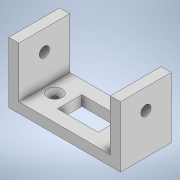
# Autodesk Inventor part: 2nd to 3rd arm linking clamp
Saved by Autodesk Inventor 2022 (Build 260153000, 153)
## iProperties
Created: 2021-06-29
Part Number: 2nd to 3rd arm linking clamp
Material: Generic
Document SubType Name: Modeling
Designer: USER
Density: 1 g/cm^3
Appearance: Default
Author: USER
Autodesk Inventor part; units mm, degrees
ref_plane "YZ Plane" through (0, 0, 0) normal (1, 0, 0) x (0, 1, 0)
ref_plane "XZ Plane" through (0, 0, 0) normal (0, 1, 0) x (-1, 0, 0)
ref_plane "XY Plane" through (0, 0, 0) normal (0, 0, 1) x (1, 0, 0)
sketch "Sketch1" plane through (0, 0, 0) normal (0, 0, 1) x (1, 0, 0)
  line L0 (0, 0) -> (55, 0)
  line L1 (55, 0) -> (55, 30)
  line L2 (55, 30) -> (50, 30)
  line L3 (50, 30) -> (50, 5)
  line L4 (50, 5) -> (5, 5)
  line L5 (5, 5) -> (5, 30)
  line L6 (5, 30) -> (0, 30)
  line L7 (0, 30) -> (0, 0)
  dimension "d0" = 55
  dimension "d1" = 30
  dimension "d2" = 5
  dimension "d3" = 25
  dimension "d4" = 45
  dimension "d5" = 25
  dimension "d6" = 5
  constraints: 16 end point, 3 perpendicular, 2 point on line, 1 horizontal, 1 vertical
  measures "d0" distance of L0.start L0.end
  measures "d1" distance of L0.end L1.end
  measures "d2" distance of L1.end L2.end
  measures "d3" distance of L2.end L3.end
  measures "d4" distance of L3.end L4.end
  measures "d5" distance of L4.end L5.end
  measures "d6" distance of L5.end L6.end
extrude "Extrusion1" add sketch "Sketch1" along normal blind 25
sketch "Sketch2" plane through (55, 0, 0) normal (1, 0, 0) x (0, 0, -1)
  circle A0 centre (-12.5, 20) radius 2.5
  line L0 (0, 30) -> (-25, 30) projected
  line L1 (0, 0) -> (0, 30) projected
  dimension "d9" = 5
  dimension "d10" = 10
  dimension "d11" = 12.5
  constraints: 1 centre point
  measures "d9" diameter of A0
  measures "d10" distance from line of L0 A0.centre
  measures "d11" distance from line of L1 A0.centre
extrude "Extrusion2" cut sketch "Sketch2" against normal through all
sketch "Sketch3" plane through (5, 5, 0) normal (0, 1, 0) x (1, 0, 0)
  line L0 (12.5, -6.5) -> (32.5, -6.5)
  line L1 (32.5, -6.5) -> (32.5, -18.5)
  line L2 (32.5, -18.5) -> (12.5, -18.5)
  line L3 (12.5, -18.5) -> (12.5, -6.5)
  line L4 (12.5, -6.5) -> (32.5, -18.5) construction
  line L5 (32.5, -6.5) -> (12.5, -18.5) construction
  line L6 (45, 0) -> (0, 0) projected
  line L7 (0, 0) -> (0, -25) projected
  point P0 (-5, 0)
  point P1 (22.5, -12.5)
  dimension "d14" = 20
  dimension "d15" = 12
  dimension "d16" = 12.5
  dimension "d17" = 22.5
  constraints: 12 end point, 2 midpoint, 2 parallel, 1 horizontal, 1 perpendicular
  measures "d14" distance of L1.end L2.end
  measures "d15" distance of L0.end L1.end
  measures "d16" distance from line of L6 point (22.5, -12.5)
  measures "d17" distance from line of L7 point (22.5, -12.5)
extrude "Extrusion3" cut sketch "Sketch3" against normal through all
sketch "Sketch4" plane through (5, 5, 0) normal (0, 1, 0) x (1, 0, 0)
  circle A0 centre (5.25, -12.5) radius 3.625
  circle A1 centre (39.75, -12.5) radius 3.625
  line L0 (0, -10) -> (0, -15) projected
  line L1 (45, 0) -> (45, -25) projected
  line L2 (45, -25) -> (0, -25) projected
  point P0 (-5, 0)
  dimension "d20" = 7.25
  dimension "d21" = 7.25
  dimension "d22" = 5.25
  dimension "d23" = 5.25
  dimension "d24" = 12.5
  dimension "d25" = 12.5
  constraints: 2 centre point
  measures "d20" diameter of A0
  measures "d21" diameter of A1
  measures "d22" distance from line of L0 A0.centre
  measures "d23" distance from line of L1 A1.centre
  measures "d24" distance from line of L2 A0.centre
  measures "d25" distance from line of L2 A1.centre
extrude "Extrusion4" cut sketch "Sketch4" against normal blind 2.1735 draft -45
sketch "Sketch5" plane through (10.25, 2.8265, 12.5) normal (0, 1, 0) x (1, 0, 0)
  circle A0 centre (0, 0) radius 1.4515
  circle A1 centre (34.5, 0) radius 1.4515
  line L0 (39.75, 12.5) -> (39.75, -12.5) projected
  point P0 (-10.25, 12.5)
  dimension "d28" = 2.903
  dimension "d29" = 2.903
  dimension "d30" = 5.25
  constraints: 2 centre point
  measures "d28" diameter of A0
  measures "d29" diameter of A1
  measures "d30" distance from line of L0 A1.centre
extrude "Extrusion5" cut sketch "Sketch5" against normal through all
body "Solid1"
